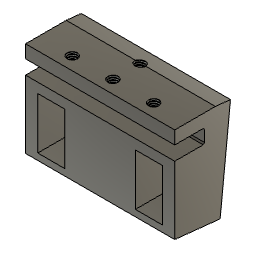
DCV Clip v5 (Autodesk Fusion 360 design; units mm, degrees)
Autodesk Fusion 360 part; units mm, degrees
sketch "Profile" plane through (0, 0, 0) normal (1, 0, 0) x (0, 1, 0) in component "Component"
  line L0 (0, 0) -> (-2.6132, 24.863)
  line L1 (0, 0) -> (-25, 0) construction
  line L2 (-2.6132, 24.863) -> (-3.6585, 34.8083)
  line L3 (-2.6132, 24.863) -> (7.332, 25.9083)
  line L4 (-2.6132, 24.863) -> (-3.1568, 30.0346)
  line L5 (-3.1568, 30.0346) -> (6.7885, 31.0798)
  line L6 (6.7885, 31.0798) -> (7.332, 25.9083)
  line L7 (-3.6585, 34.8083) -> (11.2593, 36.3762)
  line L8 (11.2593, 36.3762) -> (14.9178, 1.5679)
  line L9 (14.9178, 1.5679) -> (0, 0)
  line L10 (6.8434, 30.5572) -> (6.8434, 20.5572)
  line L11 (6.8434, 20.5572) -> (6.8434, 3.0572)
  line L12 (6.8434, 3.0572) -> (1.8434, 3.0572)
  line L13 (6.8434, 20.5572) -> (1.8434, 20.5572)
  line L14 (1.8434, 20.5572) -> (1.8434, 3.0572)
  line L15 (6.8434, 20.5572) -> (16.8434, 20.5572)
  line L16 (6.8434, 3.0572) -> (16.8434, 3.0572)
  line L17 (16.8434, 3.0572) -> (16.8434, 20.5572)
  line L18 (16.8434, 3.0572) -> (16.8434, 0)
  line L19 (16.8434, 0) -> (0, 0)
  line L20 (16.8434, 20.5572) -> (16.8434, 36.3762)
  line L21 (16.8434, 36.3762) -> (11.2593, 36.3762)
  dimension "d1" = 84
  dimension "d8" = 15
  dimension "d12" = 10
  dimension "d13" = 17.5
  dimension "d14" = 5
  dimension "d15" = 5
  dimension "d16" = 10
  dimension "d17" = 10
  constraint coincident L0.start L1.start
  constraint horizontal L1
  constraint parallel L0 L2
  constraint perpendicular L2 L3
  constraint perpendicular L3 L4
  constraint perpendicular L4 L5
  constraint perpendicular L2 L7
  constraint perpendicular L7 L8
  constraint coincident L6 L10.start
  constraint vertical L10
  constraint parallel L10 L11
  constraint perpendicular L11 L12
  constraint perpendicular L10 L13
  constraint perpendicular L11 L15
  constraint perpendicular L11 L16
  constraint perpendicular L16 L18
  constraint perpendicular L18 L19
  constraint perpendicular L15 L20
  constraint horizontal L21
  measures "d1" angle of L0 L1
  measures "d8" distance of L2.end L7.end
  measures "d12" distance of L10.start L10.end
  measures "d13" distance of L10.end L11.end
  measures "d14" distance of L11.end L12.end
  measures "d15" distance of L10.end L13.end
  measures "d16" distance of L10.end L15.end
  measures "d17" distance of L11.end L16.end
extrude "Extrude1" add sketch "Profile" along normal mid plane 20 contours L8 L15 L16 L17 makes body 1 in component "Component"
sketch "Sketch3" plane through (0, 16.8434, 0) normal (0, 1, 0) x (-1, 0, 0) in component "Component"
  line L0 (10, 20.5572) -> (-10, 20.5572)
  line L1 (-10, 20.5572) -> (-10, 3.0572)
  line L2 (-10, 3.0572) -> (10, 3.0572)
  line L3 (10, 3.0572) -> (10, 20.5572)
  line L4 (0, 20.5572) -> (0, 11.8072)
  circle A0 centre (0, 11.8072) radius 8.75
  dimension "d20" = 8.75
  dimension "d21" = 17.5
  constraint midpoint L0 L4.start
  constraint perpendicular L2 L4
  constraint coincident L4.end A0.centre
  measures "d20" distance of L4.start L4.end
  measures "d21" diameter of A0
delete_body "RemoveBody1" bodies 1 in component "Component"
extrude "Extrude2" add sketch "Profile" along normal mid plane 55 separate body contours L0 L3 L8 L9 L10 L12 L13 L14 L16 | L8 L9 L16 L18 L19 | L2 L3 L5 L6 L7 L8 L10 L15 | L8 L11 L15 L16 | L8 L15 L16 L17 | L11 L12 L13 L14 | L8 L15 L20 L21 makes body 2 in component "Component"
extrude "Extrude3" cut sketch "Sketch3" against normal blind 15 contours A0 bodies 2 in component "Component"
sketch "Sketch4" plane through (0, -3.6585, 34.8083) normal (0, -0.104528, 0.994522) x (1, 0, 0) in component "Component"
  line L0 (-27.5, 0) -> (27.5, 0)
  line L1 (27.5, 0) -> (27.5, 15)
  line L2 (27.5, 15) -> (-27.5, 15)
  line L3 (-27.5, 15) -> (-27.5, 0)
  line L4 (0, 0) -> (0, 5)
  line L5 (0, 5) -> (15, 5)
  line L6 (0, 5) -> (-15, 5)
  constraint coincident L4.start origin
  constraint perpendicular L0 L4
  constraint perpendicular L1 L5
  constraint perpendicular L4 L6
hole "Hole1" at (-15, 1.3141, 35.3309) at (0, 1.3141, 35.3309) at (15, 1.3141, 35.3309) direction (0, 0.104528, -0.994522) diameter 3.416 depth 8 tip angle 118 bodies 2 in component "Component"
thread "Thread1" "ANSI Unified Screw Threads 0.164(#8) 8-32 UNC 2B" major diameter 4.1656 minor diameter 3.4163 pitch 0.7937 angle 60 modelled right hand crest width 0.2341 on face at (-14.9149, -0.2152, 33.5614) crest through (-13.2919, 1.3349, 35.1336) on face at (0.0851, -0.2152, 33.5614) crest through (1.7082, 1.3349, 35.1336) on face at (15.0851, -0.2152, 33.5614) crest through (16.7082, 1.3349, 35.1336) on bodies 2 in component "Component"
hole "Hole2" at (0, 11.2593, 36.3762) direction (0, 0, -1) diameter 3.416 depth 20 tip angle 118 bodies 2 in component "Component"
thread "Thread2" "ANSI Unified Screw Threads 0.164(#8) 8-32 UNC 2B" major diameter 4.1656 minor diameter 3.4163 pitch 0.7937 angle 60 modelled right hand crest width 0.2341 on face at (-1.6664, 11.6338, 31.0497) crest through (1.7082, 11.2593, 36.1778) on bodies 2 in component "Component"
extrude "Extrude4" cut 1 faces at (9.1667, 7.1508, 27.6322) along direction (0, 0.994522, 0.104528) blind 1 on bodies 2 bodies 2 in component "Component"
move_body "Move1" bodies 2 to x (1, 0, 0) y (0, 0.994522, -0.104528) z (0, 0.104528, 0.994522) at (0, -0.02, -0.3824) in component "Component"
chamfer "Chamfer2" distance 0.5 angle 45 2 edges at (0, 10.98, 24.6176) (0, 10.98, 29.8176) on bodies 2 in component "Component"
sketch "Sketch5" plane through (0, 1.8532, -0.1948) normal (0, 0.994522, -0.104528) x (-1, 0, 0) in component "Component"
  circle A0 centre (0, 11.4248) radius 8.75
  line L0 (0, 11.4248) -> (-11, 11.4248)
  line L1 (-11, 11.4248) -> (-6.9602, 16.7274)
  line L2 (-11, 11.4248) -> (-6.9602, 6.1222)
  constraint coincident A0.centre L0.start
  constraint horizontal L0
  constraint coincident A0 L1.end
  constraint tangent A0 L1
  constraint coincident A0 L2.end
  constraint tangent A0 L2
extrude "Extrude5" cut sketch "Sketch5" along normal blind 500 contours A0 L0 L1 | A0 L0 L2 bodies 2 in component "Component"
chamfer "Chamfer3" distance 1 angle 45 3 edges at (8.9801, 18.2424, 12.2363) (-8.75, 17.9653, 9.5995) (8.9801, 17.6881, 6.9627) on bodies 2 in component "Component"
sketch "Sketch6" plane through (0, 0, 0) normal (0, 1, 0) x (1, 0, 0) in component "Component"
  line L0 (23, -21) -> (13, -21)
  line L1 (13, -21) -> (13, -2)
  line L2 (13, -2) -> (23, -2)
  line L3 (23, -2) -> (23, -21)
  line L4 (0, -21) -> (0, -11)
  line L5 (0, -3.0572) -> (0, -20.5572)
  line L6 (-23, -2) -> (-23, -21)
  line L7 (-23, -21) -> (-13, -21)
  line L8 (-13, -2) -> (-23, -2)
  line L9 (-13, -21) -> (-13, -2)
  constraint horizontal L0
  constraint vertical L1
  constraint horizontal L2
  constraint vertical L3
  constraint vertical L4
  constraint symmetric L0.start L5 L6.end
  constraint symmetric L0.end L5 L7.end
  constraint symmetric L1.end L5 L8.start
  constraint symmetric L2.end L5 L6.start
extrude "Extrude6" cut sketch "Sketch6" along normal mid plane 200 bodies 2 in component "Component"
component "Component" placed x (1, 0, 0) y (0, 1, 0) z (0, 0, 1) at (0, 0, 0)
named bodies: "FH DCV Clip"
